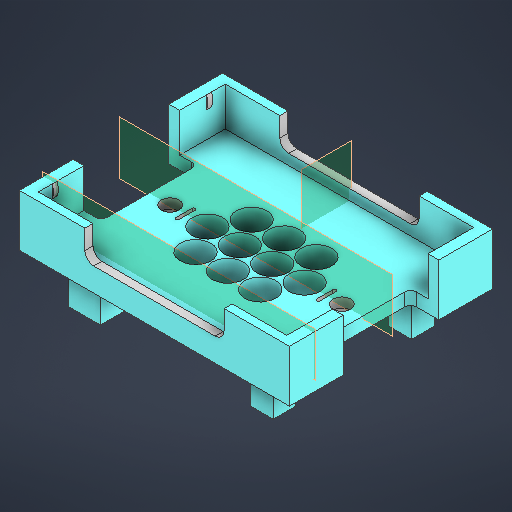
# Autodesk Inventor part: PILLARSCELLCASE18650
Saved by Autodesk Inventor 2026.2 (Build 302298000, 298)
## iProperties
Created: 2024-11-21
Part Number: PILLARSCELLCASE18650
Material: Generic
Document SubType Name: Modeling
Designer: cbast
Density: 1 g/cm^3
Appearance: Default
Mass: 190.937 g
Surface Area: 666.623 cm^2
Volume: 190.937 cm^3
Author: cbast
## iProperties of the stored document BatteryCasev1_3DPrint.ipt
Created: 2025-01-30
Part Number: BatteryCasev1_3DPrint
Material: Generic
Document SubType Name: Modeling
Designer: cbast
Density: 1 g/cm^3
Appearance: Default
Author: cbast
Autodesk Inventor part; units mm, degrees
(part 1 of 2)
ref_plane "YZ Plane" through (0, 0, 0) normal (1, 0, 0) x (0, 1, 0)
ref_plane "XZ Plane" through (0, 0, 0) normal (0, 1, 0) x (-1, 0, 0)
ref_plane "XY Plane" through (0, 0, 0) normal (0, 0, 1) x (1, 0, 0)
sketch "Sketch1" plane through (0, 0, 0) normal (0, 1, 0) x (-1, 0, 0)
  circle A0 centre (0, 0) radius 9.5
  circle A1 centre (20, 0) radius 9.5
  circle A2 centre (-20, 0) radius 9.5
  circle A3 centre (-10, 17.3205) radius 9.5
  circle A4 centre (10, 17.3205) radius 9.5
  circle A5 centre (30, 17.3205) radius 9.5
  circle A6 centre (10, -17.3205) radius 9.5
  circle A7 centre (30, -17.3205) radius 9.5
  circle A8 centre (-10, -17.3205) radius 9.5
  circle A9 centre (40, 0) radius 9.5
  line L0 (0, 0) -> (-32.9562, 0) construction
  line L1 (-32.9562, 0) -> (61.076, 0) construction
  circle A10 centre (0, 0) radius 10.5 construction
  circle A11 centre (-20, 0) radius 10.5 construction
  circle A12 centre (-10, -17.3205) radius 10.5 construction
  circle A13 centre (10, -17.3205) radius 10.5 construction
  circle A14 centre (30, -17.3205) radius 10.5 construction
  circle A15 centre (40, 0) radius 10.5 construction
  circle A16 centre (20, 0) radius 10.5 construction
  circle A17 centre (30, 17.3205) radius 10.5 construction
  circle A18 centre (10, 17.3205) radius 10.5 construction
  circle A19 centre (-10, 17.3205) radius 10.5 construction
  circle A20 centre (40, 0) radius 11.5 construction
  circle A21 centre (30, -17.3205) radius 11.5 construction
  circle A22 centre (10, -17.3205) radius 11.5 construction
  circle A23 centre (-10, -17.3205) radius 11.5 construction
  circle A24 centre (-20, 0) radius 11.5 construction
  circle A25 centre (-10, 17.3205) radius 11.5 construction
  circle A26 centre (10, 17.3205) radius 11.5 construction
  circle A27 centre (30, 17.3205) radius 11.5 construction
  circle A28 centre (0, 0) radius 11.5 construction
  circle A29 centre (20, 0) radius 11.5 construction
  arc A30 (39.9181, -11.4997) -> (39.9181, 11.4997) centre (39.9181, 0) ccw
  arc A31 (39.9181, 11.4997) -> (20, 22.9994) centre (30, 17.3205) ccw
  arc A32 (20, 22.9994) -> (0, 22.9994) centre (10, 17.3205) ccw
  arc A33 (0, 22.9994) -> (-19.9181, 11.4997) centre (-10, 17.3205) ccw
  arc A34 (-19.9181, 11.4997) -> (-19.9181, -11.4997) centre (-20, 0) ccw
  arc A35 (-19.9181, -11.4997) -> (0, -22.9994) centre (-10, -17.3205) ccw
  arc A36 (0, -22.9994) -> (20, -22.9994) centre (10, -17.3205) ccw
  arc A37 (20, -22.9994) -> (39.9181, -11.4997) centre (30, -17.3205) ccw
  point P0 (28.893, 7.4235)
  dimension "d0" = 19
  dimension "d2" = 19
  dimension "d4" = 19
  dimension "d6" = 19
  dimension "d8" = 19
  dimension "d10" = 19
  dimension "d11" = 19
  dimension "d13" = 19
  dimension "d14" = 19
  dimension "d53" = 19
  dimension "d91" = 1
  dimension "d144" = 21
  dimension "d145" = 21
  dimension "d146" = 21
  dimension "d147" = 21
  dimension "d148" = 21
  dimension "d149" = 21
  dimension "d150" = 21
  dimension "d151" = 21
  dimension "d152" = 21
  dimension "d153" = 21
  dimension "d154" = 23
  dimension "d155" = 23
  dimension "d156" = 23
  dimension "d157" = 23
  dimension "d158" = 23
  dimension "d159" = 23
  dimension "d160" = 23
  dimension "d161" = 23
  dimension "d162" = 23
  dimension "d163" = 23
  constraints: 38 centre point, 32 point on circle, 22 coincident, 16 tangent, 9 concentric, 4 end point, 2 point on line, 1 horizontal
  measures "d0" diameter of A0
  measures "d2" diameter of A1
  measures "d4" diameter of A2
  measures "d6" diameter of A3
  measures "d8" diameter of A4
  measures "d10" diameter of A5
  measures "d11" diameter of A6
  measures "d13" diameter of A7
  measures "d14" diameter of A8
  measures "d53" diameter of A9
  measures "d144" diameter of A10
  measures "d145" diameter of A11
  measures "d146" diameter of A12
  measures "d147" diameter of A13
  measures "d148" diameter of A14
  measures "d149" diameter of A15
  measures "d150" diameter of A16
  measures "d151" diameter of A17
  measures "d152" diameter of A18
  measures "d153" diameter of A19
  measures "d154" diameter of A20
  measures "d155" diameter of A21
  measures "d156" diameter of A22
  measures "d157" diameter of A23
  measures "d158" diameter of A24
  measures "d159" diameter of A25
  measures "d160" diameter of A26
  measures "d161" diameter of A27
  measures "d162" diameter of A28
  measures "d163" diameter of A29
extrude "Extrusion1" add sketch "Sketch1" along normal blind 15
sketch "Sketch4" plane through (0, 15, 0) normal (0, 1, 0) x (1, 0, 0)
  circle A0 centre (-30, 17.3205) radius 9.5 projected
  circle A1 centre (-40, 0) radius 9.5 projected
  circle A2 centre (-40, 0) radius 9.5 projected
  circle A3 centre (10, 17.3205) radius 9.5 projected
  circle A4 centre (-30, 17.3205) radius 9.5 projected
  circle A5 centre (-10, 17.3205) radius 9.5 projected
  circle A6 centre (-30, -17.3205) radius 9.5 projected
  circle A7 centre (-10, -17.3205) radius 9.5 projected
  circle A8 centre (10, -17.3205) radius 9.5 projected
  circle A9 centre (20, 0) radius 9.5 projected
  circle A10 centre (-20, 0) radius 9.5 projected
  circle A11 centre (0, 0) radius 9.5 projected
  line L0 (0, 0) -> (-10, 0) construction
  line L1 (-86.7, 57.7) -> (66.7, 57.7)
  line L2 (66.7, 57.7) -> (66.7, -57.7)
  line L3 (66.7, -57.7) -> (-86.7, -57.7)
  line L4 (-86.7, -57.7) -> (-86.7, 57.7)
  line L5 (-86.7, 57.7) -> (66.7, -57.7) construction
  line L6 (66.7, 57.7) -> (-86.7, -57.7) construction
  arc A12 (0, 22.9994) -> (-20, 22.9994) centre (-10, 17.3205) ccw projected
  arc A13 (19.9181, 11.4997) -> (0, 22.9994) centre (10, 17.3205) ccw projected
  arc A14 (19.9181, -11.4997) -> (19.9181, 11.4997) centre (20, 0) ccw projected
  arc A15 (0, -22.9994) -> (19.9181, -11.4997) centre (10, -17.3205) ccw projected
  arc A16 (-20, -22.9994) -> (0, -22.9994) centre (-10, -17.3205) ccw projected
  arc A17 (-39.9181, -11.4997) -> (-20, -22.9994) centre (-30, -17.3205) ccw projected
  circle A18 centre (-30, 17.3205) radius 11.5 construction
  arc A19 (-39.9181, 11.4997) -> (-39.9181, -11.4997) centre (-39.9181, 0) ccw projected
  arc A20 (-20, 22.9994) -> (-39.9181, 11.4997) centre (-30, 17.3205) ccw projected
  arc A21 (0, 22.9994) -> (-20, 22.9994) centre (-10, 17.3205) ccw
  arc A22 (19.9181, 11.4997) -> (0, 22.9994) centre (10, 17.3205) ccw
  arc A23 (19.9181, -11.4997) -> (19.9181, 11.4997) centre (20, 0) ccw
  arc A24 (0, -22.9994) -> (19.9181, -11.4997) centre (10, -17.3205) ccw
  arc A25 (-20, -22.9994) -> (0, -22.9994) centre (-10, -17.3205) ccw
  arc A26 (-39.9181, -11.4997) -> (-20, -22.9994) centre (-30, -17.3205) ccw
  arc A27 (-39.9181, 11.4997) -> (-39.9181, -11.4997) centre (-39.9181, 0) ccw
  arc A28 (-20, 22.9994) -> (-39.9181, 11.4997) centre (-30, 17.3205) ccw
  line L7 (-10.5, 0) -> (-9.5, 0) construction
  point P0 (-17.0502, -21.4927)
  point P1 (-17.0502, -11.5134)
  point P2 (-17.0502, -8.8009)
  point P3 (-17.0502, 8.8009)
  point P4 (-17.0502, 11.5134)
  point P5 (-17.0502, 21.4927)
  point P6 (-2.0059, 21.4927)
  point P7 (-2.0059, -11.5134)
  point P8 (-2.0059, -8.8009)
  point P9 (-2.0059, 8.8009)
  point P10 (-2.0059, 11.5134)
  point P11 (-2.0059, -21.4927)
  point P12 (-86.7, 0)
  point P13 (66.7, 0)
  dimension "d104" = 153.4
  dimension "d164" = 115.4
  dimension "d233" = 76.7
  dimension "d234" = 76.7
  constraints: 16 end point, 16 point on circle, 8 centre point, 8 concentric, 5 midpoint, 2 horizontal, 2 parallel, 1 perpendicular, 1 point on line, 4 other
  measures "d104" distance of L2.end L3.end
  measures "d164" distance of L1.end L2.end
  measures "d233" distance of point (-86.7, 0) L0.end
  measures "d234" distance of point (66.7, 0) L0.end
extrude "Extrusion7" add sketch "Sketch4" against normal blind 8 contours L1 L2 L3 L4
sketch "Sketch5" plane through (0, 15, 0) normal (0, 1, 0) x (1, 0, 0)
  line L0 (-86.7, -57.7) -> (66.7, -57.7) projected
  line L1 (66.7, -57.7) -> (66.7, 57.7) projected
  line L2 (66.7, 57.7) -> (-86.7, 57.7) projected
  line L3 (-86.7, 57.7) -> (-86.7, -57.7) projected
  circle A0 centre (-40, 0) radius 9.5 projected
  circle A1 centre (10, 17.3205) radius 9.5 projected
  circle A2 centre (-30, 17.3205) radius 9.5 projected
  circle A3 centre (-10, 17.3205) radius 9.5 projected
  circle A4 centre (-30, -17.3205) radius 9.5 projected
  circle A5 centre (-10, -17.3205) radius 9.5 projected
  circle A6 centre (10, -17.3205) radius 9.5 projected
  circle A7 centre (20, 0) radius 9.5 projected
  circle A8 centre (-20, 0) radius 9.5 projected
  circle A9 centre (0, 0) radius 9.5 projected
  line L4 (-86.7, 57.7) -> (66.7, 57.7)
  line L5 (66.7, 57.7) -> (66.7, -57.7)
  line L6 (66.7, -57.7) -> (-86.7, -57.7)
  line L7 (-86.7, -57.7) -> (-86.7, 57.7)
  line L8 (-93.3464, -62.7) -> (73.3464, -62.7)
  line L9 (73.3464, -62.7) -> (73.3464, 62.7)
  line L10 (73.3464, 62.7) -> (-93.3464, 62.7)
  line L11 (-93.3464, 62.7) -> (-93.3464, -62.7)
  line L12 (-93.3464, -62.7) -> (73.3464, 62.7) construction
  line L13 (73.3464, -62.7) -> (-93.3464, 62.7) construction
  point P0 (66.922, -57.45)
  point P1 (-10, 0)
  dimension "d169" = 5
  dimension "d170" = 6.6464
  dimension "d171" = 166.6929
  dimension "d172" = 125.4
  dimension "d221" = 6.6464
  constraints: 20 end point, 4 parallel, 4 point on line, 2 horizontal, 2 midpoint, 2 perpendicular
  measures "d169" distance between parallel lines of L10 L4
  measures "d170" distance between parallel lines of L9 L5
  measures "d171" distance of L9.end L10.end
  measures "d172" distance of L10.end L8.start
  measures "d221" distance between parallel lines of L3 L11
extrude "Extrusion8" add sketch "Sketch5" along normal blind 24 and the other way blind 8 contours L11 L10 L9 L8
sketch "Sketch6" plane through (0, 15, 0) normal (0, 1, 0) x (1, 0, 0)
  line L0 (59.472, 57.1514) -> (59.472, 25.95) construction
  line L1 (59.472, 25.95) -> (66.7, 25.95) construction
  line L2 (-79.472, -57.7) -> (-79.472, -25.95) construction
  line L3 (-79.472, -25.95) -> (-86.7, -25.95) construction
  circle A0 centre (59.472, 25.95) radius 3.615
  circle A1 centre (59.472, -25.95) radius 3.615
  circle A2 centre (-79.472, -25.95) radius 3.615
  circle A3 centre (-79.472, 25.95) radius 3.615
  line L4 (73.3464, -62.7) -> (73.3464, 62.7) projected
  line L5 (73.3464, 62.7) -> (-93.3464, 62.7) projected
  line L6 (-93.3464, 62.7) -> (-93.3464, -62.7) projected
  line L7 (-93.3464, -62.7) -> (73.3464, -62.7) projected
  line L8 (-86.7, -57.7) -> (-86.7, 57.7) projected
  line L9 (-86.7, 57.7) -> (66.7, 57.7) projected
  line L10 (66.7, 57.7) -> (66.7, -57.7) projected
  line L11 (66.7, -57.7) -> (-86.7, -57.7) projected
  line L12 (-86.7, -57.7) -> (66.7, -57.7) projected
  line L13 (66.7, -57.7) -> (66.7, 57.7) projected
  line L14 (66.7, 57.7) -> (-86.7, 57.7) projected
  line L15 (-86.7, 57.7) -> (-86.7, -57.7) projected
  circle A4 centre (-40, 0) radius 9.5 projected
  circle A5 centre (10, 17.3205) radius 9.5 projected
  circle A6 centre (-30, 17.3205) radius 9.5 projected
  circle A7 centre (-10, 17.3205) radius 9.5 projected
  circle A8 centre (-30, -17.3205) radius 9.5 projected
  circle A9 centre (-10, -17.3205) radius 9.5 projected
  circle A10 centre (10, -17.3205) radius 9.5 projected
  circle A11 centre (20, 0) radius 9.5 projected
  circle A12 centre (-20, 0) radius 9.5 projected
  circle A13 centre (0, 0) radius 9.5 projected
  line L16 (-86.7, 57.7) -> (66.7, 57.7)
  line L17 (66.7, 57.7) -> (66.7, -57.7)
  line L18 (66.7, -57.7) -> (-86.7, -57.7)
  line L19 (-86.7, -57.7) -> (-86.7, 57.7)
  dimension "d123" = 7.23
  dimension "d124" = 7.23
  dimension "d125" = 7.23
  dimension "d140" = 7.23
  dimension "d179" = 31.75
  dimension "d180" = 7.228
  dimension "d181" = 7.228
  dimension "d182" = 31.75
  dimension "d183" = 31.75
  dimension "d184" = 7.228
  dimension "d185" = 7.228
  dimension "d186" = 31.75
  constraints: 16 end point, 4 centre point, 2 coincident, 2 parallel, 1 horizontal, 1 perpendicular
  measures "d123" diameter of A0
  measures "d124" diameter of A1
  measures "d125" diameter of A2
  measures "d140" diameter of A3
  measures "d179" distance from line of A3.centre L16
  measures "d180" distance from line of A3.centre L15
  measures "d181" distance from line of A2.centre L8
  measures "d182" distance from line of L2.end L18
  measures "d183" distance from line of L12 A1.centre
  measures "d184" distance from line of L17 A1.centre
  measures "d185" distance from line of L17 L0.end
  measures "d186" distance from line of L16 L0.end
extrude "Extrusion6" cut sketch "Sketch6" against normal through all contours A0 | A1 | A2 | A3
sketch "Sketch7" plane through (-93.3464, 7, 62.7) normal (-1, 0, 0) x (0, 0, 1)
  line L0 (-120.4, 8) -> (-5, 8) projected
  line L1 (0, 0) -> (-125.4, 0) projected
  line L2 (-125.4, 32) -> (0, 32) projected
  line L3 (-92.265, 8) -> (-85.035, 8) projected
  line L4 (-40.365, 8) -> (-33.135, 8) projected
  line L5 (-92.265, 8) -> (-33.135, 8)
  line L6 (-33.135, 8) -> (-33.135, 32)
  line L7 (-33.135, 32) -> (-92.265, 32)
  line L8 (-92.265, 32) -> (-92.265, 8)
  point P0 (-62.7, -7)
  point P1 (-92.265, 32)
  constraints: 8 end point, 2 parallel, 1 horizontal, 1 perpendicular, 1 point on line
extrude "Extrusion9" cut sketch "Sketch7" against normal through all
sketch "Sketch10" plane through (0, 7, 0) normal (0, -1, 0) x (1, 0, 0)
  circle A0 centre (-79.472, 25.95) radius 3.615 projected
  circle A1 centre (59.472, 25.95) radius 3.615 projected
  circle A2 centre (-79.472, -25.95) radius 3.615 projected
  circle A3 centre (59.472, -25.95) radius 3.615 projected
  line L0 (73.3464, -62.7) -> (73.3464, 62.7) projected
  line L1 (73.3464, 62.7) -> (-93.3464, 62.7) projected
  line L2 (-93.3464, 62.7) -> (-93.3464, -62.7) projected
  line L3 (-93.3464, -62.7) -> (73.3464, -62.7) projected
  arc A4 (-39.9181, -11.4997) -> (-20, -22.9994) centre (-30, -17.3205) ccw projected
  arc A5 (-39.9181, 11.4997) -> (-39.9181, -11.4997) centre (-39.9181, 0) ccw projected
  arc A6 (-20, 22.9994) -> (-39.9181, 11.4997) centre (-30, 17.3205) ccw projected
  arc A7 (0, 22.9994) -> (-20, 22.9994) centre (-10, 17.3205) ccw projected
  arc A8 (19.9181, 11.4997) -> (0, 22.9994) centre (10, 17.3205) ccw projected
  arc A9 (19.9181, -11.4997) -> (19.9181, 11.4997) centre (20, 0) ccw projected
  arc A10 (0, -22.9994) -> (19.9181, -11.4997) centre (10, -17.3205) ccw projected
  arc A11 (-20, -22.9994) -> (0, -22.9994) centre (-10, -17.3205) ccw projected
  line L4 (-93.3464, 62.7) -> (-63.3464, 62.7) construction
  line L5 (-93.3464, 62.7) -> (-93.3464, 42.7) construction
  line L6 (-93.3464, 42.7) -> (-63.3464, 42.7) construction
  line L7 (-73.3464, 52.7) -> (-53.3464, 52.7)
  line L8 (-53.3464, 52.7) -> (-53.3464, 32.7)
  line L9 (-53.3464, 32.7) -> (-73.3464, 32.7)
  line L10 (-73.3464, 32.7) -> (-73.3464, 52.7)
  line L11 (-73.3464, 52.7) -> (-53.3464, 32.7) construction
  line L12 (-53.3464, 52.7) -> (-73.3464, 32.7) construction
  line L13 (-70.8464, 50.2) -> (-55.8464, 50.2)
  line L14 (-55.8464, 50.2) -> (-55.8464, 35.2)
  line L15 (-55.8464, 35.2) -> (-70.8464, 35.2)
  line L16 (-70.8464, 35.2) -> (-70.8464, 50.2)
  line L17 (-70.8464, 50.2) -> (-55.8464, 35.2) construction
  line L18 (-55.8464, 50.2) -> (-70.8464, 35.2) construction
  line L19 (-93.3464, 0) -> (73.3464, 0) construction
  line L20 (-73.3464, -52.7) -> (-53.3464, -52.7)
  line L21 (-53.3464, -52.7) -> (-53.3464, -32.7)
  line L22 (-53.3464, -32.7) -> (-73.3464, -32.7)
  line L23 (-73.3464, -32.7) -> (-73.3464, -52.7)
  line L24 (-73.3464, -52.7) -> (-53.3464, -32.7) construction
  line L25 (-53.3464, -52.7) -> (-73.3464, -32.7) construction
  line L26 (-70.8464, -50.2) -> (-55.8464, -50.2)
  line L27 (-55.8464, -50.2) -> (-55.8464, -35.2)
  line L28 (-55.8464, -35.2) -> (-70.8464, -35.2)
  line L29 (-70.8464, -35.2) -> (-70.8464, -50.2)
  line L30 (-70.8464, -50.2) -> (-55.8464, -35.2) construction
  line L31 (-55.8464, -50.2) -> (-70.8464, -35.2) construction
  line L32 (73.3464, 62.7) -> (43.3464, 62.7) construction
  line L33 (43.3464, 62.7) -> (43.3464, 42.7) construction
  line L34 (36.3464, 49.7) -> (50.3464, 49.7)
  line L35 (50.3464, 49.7) -> (50.3464, 35.7)
  line L36 (50.3464, 35.7) -> (36.3464, 35.7)
  line L37 (36.3464, 35.7) -> (36.3464, 49.7)
  line L38 (36.3464, 49.7) -> (50.3464, 35.7) construction
  line L39 (50.3464, 49.7) -> (36.3464, 35.7) construction
  line L40 (36.3464, -49.7) -> (50.3464, -49.7)
  line L41 (50.3464, -49.7) -> (50.3464, -35.7)
  line L42 (50.3464, -35.7) -> (36.3464, -35.7)
  line L43 (36.3464, -35.7) -> (36.3464, -49.7)
  line L44 (36.3464, -49.7) -> (50.3464, -35.7) construction
  line L45 (50.3464, -49.7) -> (36.3464, -35.7) construction
  line L46 (43.3464, -42.7) -> (43.3464, -62.7) construction
  line L47 (43.3464, -42.7) -> (73.3464, -42.7) construction
  line L48 (-63.3464, -42.7) -> (-63.3464, -62.7) construction
  line L49 (-63.3464, -42.7) -> (-93.3464, -42.7) construction
  point P0 (0, 0)
  dimension "d209" = 30
  dimension "d210" = 20
  dimension "d211" = 20
  dimension "d212" = 20
  dimension "d213" = 15
  dimension "d214" = 15
  dimension "d215" = 30
  dimension "d216" = 20
  dimension "d217" = 14
  dimension "d218" = 14
  dimension "d224" = 30
  dimension "d225" = 30
  dimension "d226" = 20
  dimension "d227" = 20
  constraints: 92 end point, 14 symmetric about line, 8 midpoint, 8 point on line, 7 parallel, 6 perpendicular, 4 horizontal
  measures "d209" distance of L1.end L4.end
  measures "d210" distance of L1.end L5.end
  measures "d211" distance of L8.end L9.end
  measures "d212" distance of L7.end L8.end
  measures "d213" distance of L14.end L15.end
  measures "d214" distance of L13.end L14.end
  measures "d215" distance of L0.end L32.end
  measures "d216" distance of L32.end L33.end
  measures "d217" distance of L35.end L36.end
  measures "d218" distance of L34.end L35.end
  measures "d224" distance of L48.start L49.end
  measures "d225" distance of L46.start L47.end
  measures "d226" distance of L46.start L46.end
  measures "d227" distance of L48.start L48.end
extrude "Extrusion11" add sketch "Sketch10" along normal blind 25 contours L7 L8 L9 L10 | L23 L22 L21 L20 | L34 L35 L36 L37 | L43 L42 L41 L40
sketch "Sketch11" plane through (0, 7, 0) normal (0, -1, 0) x (1, 0, 0)
  line L0 (-70.8464, 50.2) -> (-70.8464, 35.2) projected
  line L1 (-70.8464, 35.2) -> (-55.8464, 35.2) projected
  line L2 (-55.8464, 35.2) -> (-55.8464, 50.2) projected
  line L3 (-55.8464, 50.2) -> (-70.8464, 50.2) projected
  line L4 (-70.8464, 50.2) -> (-55.8464, 50.2)
  line L5 (-55.8464, 50.2) -> (-55.8464, 35.2)
  line L6 (-55.8464, 35.2) -> (-70.8464, 35.2)
  line L7 (-70.8464, 35.2) -> (-70.8464, 50.2)
  line L8 (-55.8464, -35.2) -> (-70.8464, -35.2) projected
  line L9 (-70.8464, -35.2) -> (-70.8464, -50.2) projected
  line L10 (-70.8464, -50.2) -> (-55.8464, -50.2) projected
  line L11 (-55.8464, -50.2) -> (-55.8464, -35.2) projected
  line L12 (-70.8464, -35.2) -> (-55.8464, -35.2)
  line L13 (-55.8464, -35.2) -> (-55.8464, -50.2)
  line L14 (-55.8464, -50.2) -> (-70.8464, -50.2)
  line L15 (-70.8464, -50.2) -> (-70.8464, -35.2)
  point P0 (0, 0)
  constraints: 16 end point, 4 parallel, 2 horizontal, 2 perpendicular
extrude "Extrusion12" add sketch "Sketch11" along normal up to surface (12.5 mm away)
sketch "Sketch13" plane through (0, 7, 0) normal (0, -1, 0) x (1, 0, 0)
  line L0 (36.3464, 35.7) -> (36.3464, 49.7) projected
  line L1 (36.3464, 49.7) -> (50.3464, 49.7) projected
  line L2 (50.3464, 49.7) -> (50.3464, 35.7) projected
  line L3 (50.3464, 35.7) -> (36.3464, 35.7) projected
  line L4 (-73.3464, -32.7) -> (-53.3464, -32.7) projected
  line L5 (-53.3464, -32.7) -> (-53.3464, -52.7) projected
  line L6 (-53.3464, -52.7) -> (-73.3464, -52.7) projected
  line L7 (-73.3464, -52.7) -> (-73.3464, -32.7) projected
  line L8 (36.3464, -49.7) -> (36.3464, -35.7) projected
  line L9 (36.3464, -35.7) -> (50.3464, -35.7) projected
  line L10 (50.3464, -35.7) -> (50.3464, -49.7) projected
  line L11 (50.3464, -49.7) -> (36.3464, -49.7) projected
  line L12 (-73.3464, 32.7) -> (-73.3464, 52.7) projected
  line L13 (-73.3464, 52.7) -> (-53.3464, 52.7) projected
  line L14 (-53.3464, 52.7) -> (-53.3464, 32.7) projected
  line L15 (-53.3464, 32.7) -> (-73.3464, 32.7) projected
  circle A0 centre (-79.472, 25.95) radius 3.615 projected
  circle A1 centre (59.472, 25.95) radius 3.615 projected
  circle A2 centre (-79.472, -25.95) radius 3.615 projected
  circle A3 centre (59.472, -25.95) radius 3.615 projected
  line L16 (73.3464, -62.7) -> (73.3464, 62.7) projected
  line L17 (73.3464, 62.7) -> (-93.3464, 62.7) projected
  line L18 (-93.3464, 62.7) -> (-93.3464, -62.7) projected
  line L19 (-93.3464, -62.7) -> (73.3464, -62.7) projected
  arc A4 (-39.9181, -11.4997) -> (-20, -22.9994) centre (-30, -17.3205) ccw projected
  arc A5 (-39.9181, 11.4997) -> (-39.9181, -11.4997) centre (-39.9181, 0) ccw projected
  arc A6 (-20, 22.9994) -> (-39.9181, 11.4997) centre (-30, 17.3205) ccw projected
  arc A7 (0, 22.9994) -> (-20, 22.9994) centre (-10, 17.3205) ccw projected
  arc A8 (19.9181, 11.4997) -> (0, 22.9994) centre (10, 17.3205) ccw projected
  arc A9 (19.9181, -11.4997) -> (19.9181, 11.4997) centre (20, 0) ccw projected
  arc A10 (0, -22.9994) -> (19.9181, -11.4997) centre (10, -17.3205) ccw projected
  arc A11 (-20, -22.9994) -> (0, -22.9994) centre (-10, -17.3205) ccw projected
  line L20 (-93.3464, 29.565) -> (-75.857, 29.565)
  line L21 (-75.857, 29.565) -> (-75.857, -29.565)
  line L22 (-75.857, -29.565) -> (-93.3464, -29.565)
  line L23 (-93.3464, -29.565) -> (-93.3464, 29.565)
  line L24 (-10, 27.2798) -> (-10, -25.95) construction
  line L25 (73.3464, 29.565) -> (55.857, 29.565)
  line L26 (55.857, 29.565) -> (55.857, -29.565)
  line L27 (55.857, -29.565) -> (73.3464, -29.565)
  circle A12 centre (-79.472, -25.95) radius 3.615 projected
  line L28 (-86.7, 29.565) -> (-86.7, 57.7) projected
  line L29 (-86.7, 57.7) -> (66.7, 57.7) projected
  line L30 (66.7, 57.7) -> (66.7, 29.565) projected
  line L31 (66.7, 29.565) -> (73.3464, 29.565) projected
  line L32 (73.3464, -29.565) -> (73.3464, 29.565) projected
  line L33 (66.7, -29.565) -> (73.3464, -29.565) projected
  line L34 (66.7, -29.565) -> (66.7, -57.7) projected
  line L35 (66.7, -57.7) -> (-86.7, -57.7) projected
  line L36 (-86.7, -57.7) -> (-86.7, -29.565) projected
  line L37 (-93.3464, -29.565) -> (-86.7, -29.565) projected
  line L38 (-93.3464, 29.565) -> (-93.3464, -29.565) projected
  line L39 (-93.3464, 29.565) -> (-86.7, 29.565) projected
  circle A13 centre (59.472, -25.95) radius 3.615 projected
  circle A14 centre (-79.472, 25.95) radius 3.615 projected
  circle A15 centre (-40, 0) radius 9.5 projected
  circle A16 centre (10, -17.3205) radius 9.5 projected
  circle A17 centre (-30, -17.3205) radius 9.5 projected
  circle A18 centre (-10, -17.3205) radius 9.5 projected
  circle A19 centre (-30, 17.3205) radius 9.5 projected
  circle A20 centre (-10, 17.3205) radius 9.5 projected
  circle A21 centre (10, 17.3205) radius 9.5 projected
  circle A22 centre (20, 0) radius 9.5 projected
  circle A23 centre (-20, 0) radius 9.5 projected
  circle A24 centre (0, 0) radius 9.5 projected
  circle A25 centre (59.472, 25.95) radius 3.615 projected
  line L40 (-10.5, 0) -> (-9.5, 0) construction
  point P0 (59.472, -29.565)
  point P1 (59.472, 29.565)
  point P2 (55.857, 25.95)
  point P3 (55.857, -25.95)
  point P4 (-79.472, -29.565)
  point P5 (-75.857, -25.95)
  point P6 (-75.857, 25.95)
  point P7 (-79.472, 29.565)
  dimension "d235" = 17.4895
  dimension "d236" = 17.4895
  constraints: 18 end point, 4 symmetric about line, 2 horizontal, 2 horizontal alignment, 2 parallel, 1 perpendicular, 1 point on line, 1 vertical, 2 other
  measures "d235" distance between parallel lines of L21 L18
  measures "d236" distance between parallel lines of L16 L26
extrude "Extrusion14" cut sketch "Sketch13" against normal blind 10 contours L21 A2 L22 L18 L20 A0 | L25 L16 L27 A3 L26 A1
sketch "Sketch15" plane through (0, 7, 0) normal (0, -1, 0) x (1, 0, 0)
  line L0 (-39.8605, 53.1473) -> (15.842, 53.1473) construction
  line L1 (15.842, 53.1473) -> (15.842, 30.1509) construction
  line L2 (15.842, 30.1509) -> (-39.8605, 30.1509) construction
  line L3 (-39.8605, 30.1509) -> (-39.8605, 53.1473) construction
  line L4 (-27.8722, 48.7866) -> (-30.2445, 48.7866)
  line L5 (-30.2445, 48.7866) -> (-30.6581, 47.8297)
  spline S0 degree 2 poles (-30.6581, 47.8297) (-30.8126, 47.4709) (-30.8126, 47.2965) knots 0 0 0 1 1 1
  spline S1 degree 2 poles (-30.8126, 47.2965) (-30.8126, 47.157) (-30.5435, 46.9427) (-30.1049, 46.9128) knots 0 0 0 1 2 2 2
  line L6 (-30.1049, 46.9128) -> (-30.1049, 46.7483)
  line L7 (-30.1049, 46.7483) -> (-32.0286, 46.7483)
  line L8 (-32.0286, 46.7483) -> (-32.0286, 46.9128)
  spline S2 degree 2 poles (-32.0286, 46.9128) (-31.6449, 46.9825) (-31.5352, 47.0872) knots 0 0 0 1 1 1
  spline S3 degree 2 poles (-31.5352, 47.0872) (-31.306, 47.3065) (-31.0269, 47.9693) knots 0 0 0 1 1 1
  line L9 (-31.0269, 47.9693) -> (-28.874, 52.9878)
  line L10 (-28.874, 52.9878) -> (-28.7145, 52.9878)
  line L11 (-28.7145, 52.9878) -> (-26.5914, 47.9145)
  spline S4 degree 2 poles (-26.5914, 47.9145) (-26.3373, 47.3015) (-25.9186, 46.9377) (-25.5449, 46.9128) knots 0 0 0 1 2 2 2
  line L12 (-25.5449, 46.9128) -> (-25.5449, 46.7483)
  line L13 (-25.5449, 46.7483) -> (-27.952, 46.7483)
  line L14 (-27.952, 46.7483) -> (-27.952, 46.9128)
  spline S5 degree 2 poles (-27.952, 46.9128) (-27.5882, 46.9327) (-27.329, 47.137) (-27.329, 47.2865) knots 0 0 0 1 2 2 2
  spline S6 degree 2 poles (-27.329, 47.2865) (-27.329, 47.4859) (-27.5084, 47.9145) knots 0 0 0 1 1 1
  line L15 (-27.5084, 47.9145) -> (-27.8722, 48.7866)
  line L16 (-28.0118, 49.1205) -> (-29.0384, 51.5874)
  line L17 (-29.0384, 51.5874) -> (-30.1049, 49.1205)
  line L18 (-30.1049, 49.1205) -> (-28.0118, 49.1205)
  line L19 (-19.2156, 46.7483) -> (-20.8453, 46.7483)
  line L20 (-20.8453, 46.7483) -> (-22.9135, 49.5989)
  spline S7 degree 2 poles (-22.9135, 49.5989) (-23.1427, 49.589) (-23.2823, 49.589) knots 0 0 0 1 1 1
  spline S8 degree 2 poles (-23.2823, 49.589) (-23.3421, 49.589) (-23.4767, 49.594) (-23.5464, 49.5989) knots 0 0 0 1 2 2 2
  line L21 (-23.5464, 49.5989) -> (-23.5464, 47.8297)
  spline S9 degree 2 poles (-23.5464, 47.8297) (-23.5464, 47.2516) (-23.4218, 47.1121) knots 0 0 0 1 1 1
  spline S10 degree 2 poles (-23.4218, 47.1121) (-23.2524, 46.9128) (-22.9135, 46.9128) knots 0 0 0 1 1 1
  line L22 (-22.9135, 46.9128) -> (-22.6743, 46.9128)
  line L23 (-22.6743, 46.9128) -> (-22.6743, 46.7483)
  line L24 (-22.6743, 46.7483) -> (-25.2807, 46.7483)
  line L25 (-25.2807, 46.7483) -> (-25.2807, 46.9128)
  line L26 (-25.2807, 46.9128) -> (-25.0515, 46.9128)
  spline S11 degree 2 poles (-25.0515, 46.9128) (-24.6677, 46.9128) (-24.5033, 47.1669) knots 0 0 0 1 1 1
  spline S12 degree 2 poles (-24.5033, 47.1669) (-24.4086, 47.3065) (-24.4086, 47.8297) knots 0 0 0 1 1 1
  line L27 (-24.4086, 47.8297) -> (-24.4086, 51.7668)
  spline S13 degree 2 poles (-24.4086, 51.7668) (-24.4086, 52.3449) (-24.5332, 52.4845) knots 0 0 0 1 1 1
  spline S14 degree 2 poles (-24.5332, 52.4845) (-24.7076, 52.6838) (-25.0515, 52.6838) knots 0 0 0 1 1 1
  line L28 (-25.0515, 52.6838) -> (-25.2807, 52.6838)
  line L29 (-25.2807, 52.6838) -> (-25.2807, 52.8483)
  line L30 (-25.2807, 52.8483) -> (-23.063, 52.8483)
  spline S15 degree 2 poles (-23.063, 52.8483) (-22.0912, 52.8483) (-21.1692, 52.5642) (-20.5263, 51.8067) (-20.5263, 51.2784) knots 0 0 0 1 2 3 3 3
  spline S16 degree 2 poles (-20.5263, 51.2784) (-20.5263, 50.7153) (-21.2589, 49.888) (-22.0314, 49.7186) knots 0 0 0 1 2 2 2
  line L31 (-22.0314, 49.7186) -> (-20.7655, 47.9693)
  spline S17 degree 2 poles (-20.7655, 47.9693) (-20.332, 47.3663) (-19.714, 46.9676) (-19.2156, 46.9128) knots 0 0 0 1 2 2 2
  line L32 (-19.2156, 46.9128) -> (-19.2156, 46.7483)
  spline S18 degree 2 poles (-23.5464, 49.883) (-23.4617, 49.883) (-23.3371, 49.878) (-23.2972, 49.878) knots 0 0 0 1 2 2 2
  spline S19 degree 2 poles (-23.2972, 49.878) (-22.4351, 49.878) (-21.5579, 50.6355) (-21.5579, 51.2186) knots 0 0 0 1 2 2 2
  spline S20 degree 2 poles (-21.5579, 51.2186) (-21.5579, 51.7918) (-22.2656, 52.5044) (-22.8487, 52.5044) knots 0 0 0 1 2 2 2
  spline S21 degree 2 poles (-22.8487, 52.5044) (-23.1079, 52.5044) (-23.5464, 52.4197) knots 0 0 0 1 1 1
  line L33 (-23.5464, 52.4197) -> (-23.5464, 49.883)
  line L34 (-13.9728, 52.8483) -> (-13.908, 51.418)
  line L35 (-13.908, 51.418) -> (-14.0775, 51.418)
  spline S22 degree 2 poles (-14.0775, 51.418) (-14.1273, 51.7918) (-14.212, 51.9562) knots 0 0 0 1 1 1
  spline S23 degree 2 poles (-14.212, 51.9562) (-14.3516, 52.2154) (-14.815, 52.4645) (-15.1938, 52.4645) knots 0 0 0 1 2 2 2
  line L36 (-15.1938, 52.4645) -> (-16.051, 52.4645)
  line L37 (-16.051, 52.4645) -> (-16.051, 47.8048)
  spline S24 degree 2 poles (-16.051, 47.8048) (-16.051, 47.2417) (-15.9314, 47.1021) knots 0 0 0 1 1 1
  spline S25 degree 2 poles (-15.9314, 47.1021) (-15.757, 46.9128) (-15.4031, 46.9128) knots 0 0 0 1 1 1
  line L38 (-15.4031, 46.9128) -> (-15.1938, 46.9128)
  line L39 (-15.1938, 46.9128) -> (-15.1938, 46.7483)
  line L40 (-15.1938, 46.7483) -> (-17.7753, 46.7483)
  line L41 (-17.7753, 46.7483) -> (-17.7753, 46.9128)
  line L42 (-17.7753, 46.9128) -> (-17.561, 46.9128)
  spline S26 degree 2 poles (-17.561, 46.9128) (-17.1723, 46.9128) (-17.0128, 47.147) knots 0 0 0 1 1 1
  spline S27 degree 2 poles (-17.0128, 47.147) (-16.9132, 47.2915) (-16.9132, 47.8048) knots 0 0 0 1 1 1
  line L43 (-16.9132, 47.8048) -> (-16.9132, 52.4645)
  line L44 (-16.9132, 52.4645) -> (-17.6458, 52.4645)
  spline S28 degree 2 poles (-17.6458, 52.4645) (-18.0744, 52.4645) (-18.2538, 52.3998) knots 0 0 0 1 1 1
  spline S29 degree 2 poles (-18.2538, 52.3998) (-18.488, 52.315) (-18.8169, 51.8316) (-18.8518, 51.418) knots 0 0 0 1 2 2 2
  line L45 (-18.8518, 51.418) -> (-19.0213, 51.418)
  line L46 (-19.0213, 51.418) -> (-18.9515, 52.8483)
  line L47 (-18.9515, 52.8483) -> (-13.9728, 52.8483)
  line L48 (-9.4377, 52.9878) -> (-9.4377, 50.8797)
  line L49 (-9.4377, 50.8797) -> (-9.6021, 50.8797)
  spline S30 degree 2 poles (-9.6021, 50.8797) (-9.6819, 51.4878) (-10.1055, 52.2054) (-10.878, 52.629) (-11.2966, 52.629) knots 0 0 0 1 2 3 3 3
  spline S31 degree 2 poles (-11.2966, 52.629) (-11.765, 52.629) (-12.378, 52.0559) (-12.378, 51.6921) knots 0 0 0 1 2 2 2
  spline S32 degree 2 poles (-12.378, 51.6921) (-12.378, 51.413) (-12.1837, 51.1837) knots 0 0 0 1 1 1
  spline S33 degree 2 poles (-12.1837, 51.1837) (-11.9046, 50.8449) (-10.853, 50.2817) knots 0 0 0 1 1 1
  spline S34 degree 2 poles (-10.853, 50.2817) (-10.0008, 49.8232) (-9.3729, 49.3348) (-9.034, 48.667) (-9.034, 48.3032) knots 0 0 0 1 2 3 3 3
  spline S35 degree 2 poles (-9.034, 48.3032) (-9.034, 47.6105) (-10.1105, 46.6087) (-10.9577, 46.6087) knots 0 0 0 1 2 2 2
  spline S36 degree 2 poles (-10.9577, 46.6087) (-11.2218, 46.6087) (-11.4561, 46.6486) knots 0 0 0 1 1 1
  spline S37 degree 2 poles (-11.4561, 46.6486) (-11.5956, 46.6735) (-12.4727, 46.9576) (-12.5923, 46.9576) knots 0 0 0 1 2 2 2
  spline S38 degree 2 poles (-12.5923, 46.9576) (-12.702, 46.9576) (-12.8365, 46.823) (-12.8664, 46.6087) knots 0 0 0 1 2 2 2
  line L50 (-12.8664, 46.6087) -> (-13.0309, 46.6087)
  line L51 (-13.0309, 46.6087) -> (-13.0309, 48.7019)
  line L52 (-13.0309, 48.7019) -> (-12.8664, 48.7019)
  spline S39 degree 2 poles (-12.8664, 48.7019) (-12.7518, 48.044) (-12.3531, 47.3912) (-11.5358, 46.9576) (-11.0524, 46.9576) knots 0 0 0 1 2 3 3 3
  spline S40 degree 2 poles (-11.0524, 46.9576) (-10.4892, 46.9576) (-9.8364, 47.5507) (-9.8364, 47.9593) knots 0 0 0 1 2 2 2
  spline S41 degree 2 poles (-9.8364, 47.9593) (-9.8364, 48.1836) (-10.0856, 48.6421) (-10.3447, 48.8414) knots 0 0 0 1 2 2 2
  spline S42 degree 2 poles (-10.3447, 48.8414) (-10.5191, 48.976) (-12.089, 49.8531) (-12.7518, 50.3764) (-13.0957, 51.0043) (-13.0957, 51.3831) knots 0 0 0 1 2 3 4 4 4
  spline S43 degree 2 poles (-13.0957, 51.3831) (-13.0957, 52.0409) (-12.084, 52.9878) (-11.3016, 52.9878) knots 0 0 0 1 2 2 2
  spline S44 degree 2 poles (-11.3016, 52.9878) (-10.8182, 52.9878) (-10.27, 52.7486) knots 0 0 0 1 1 1
  spline S45 degree 2 poles (-10.27, 52.7486) (-10.0158, 52.639) (-9.9111, 52.639) knots 0 0 0 1 1 1
  spline S46 degree 2 poles (-9.9111, 52.639) (-9.7965, 52.639) (-9.647, 52.7785) (-9.6021, 52.9878) knots 0 0 0 1 2 2 2
  line L53 (-9.6021, 52.9878) -> (-9.4377, 52.9878)
  line L54 (-0.9655, 48.4378) -> (-0.8159, 48.4079)
  line L55 (-0.8159, 48.4079) -> (-1.3392, 46.7483)
  line L56 (-1.3392, 46.7483) -> (-6.0588, 46.7483)
  line L57 (-6.0588, 46.7483) -> (-6.0588, 46.9128)
  line L58 (-6.0588, 46.9128) -> (-5.8295, 46.9128)
  spline S47 degree 2 poles (-5.8295, 46.9128) (-5.4458, 46.9128) (-5.2813, 47.1669) knots 0 0 0 1 1 1
  spline S48 degree 2 poles (-5.2813, 47.1669) (-5.1866, 47.3065) (-5.1866, 47.8297) knots 0 0 0 1 1 1
  line L59 (-5.1866, 47.8297) -> (-5.1866, 51.7668)
  spline S49 degree 2 poles (-5.1866, 51.7668) (-5.1866, 52.34) (-5.3112, 52.4845) knots 0 0 0 1 1 1
  spline S50 degree 2 poles (-5.3112, 52.4845) (-5.4856, 52.6838) (-5.8295, 52.6838) knots 0 0 0 1 1 1
  line L60 (-5.8295, 52.6838) -> (-6.0588, 52.6838)
  line L61 (-6.0588, 52.6838) -> (-6.0588, 52.8483)
  line L62 (-6.0588, 52.8483) -> (-3.3028, 52.8483)
  line L63 (-3.3028, 52.8483) -> (-3.3028, 52.6838)
  spline S51 degree 2 poles (-3.3028, 52.6838) (-3.7912, 52.6888) (-4.1799, 52.4994) (-4.3244, 52.2104) (-4.3244, 51.6672) knots 0 0 0 1 2 3 3 3
  line L64 (-4.3244, 51.6672) -> (-4.3244, 47.8347)
  spline S52 degree 2 poles (-4.3244, 47.8347) (-4.3244, 47.461) (-4.2547, 47.3214) knots 0 0 0 1 1 1
  spline S53 degree 2 poles (-4.2547, 47.3214) (-4.1999, 47.2267) (-3.9756, 47.137) (-3.3825, 47.137) knots 0 0 0 1 2 2 2
  line L65 (-3.3825, 47.137) -> (-2.939, 47.137)
  spline S54 degree 2 poles (-2.939, 47.137) (-2.2363, 47.137) (-1.6682, 47.3463) (-1.1997, 47.8696) (-0.9655, 48.4378) knots 0 0 0 1 2 3 3 3
  spline S55 degree 2 poles (1.9998, 47.3463) (1.3669, 46.8529) (1.2024, 46.7782) knots 0 0 0 1 1 1
  spline S56 degree 2 poles (1.2024, 46.7782) (0.9632, 46.6636) (0.6891, 46.6636) knots 0 0 0 1 1 1
  spline S57 degree 2 poles (0.6891, 46.6636) (0.2605, 46.6636) (-0.2927, 47.2467) (-0.2927, 47.7251) knots 0 0 0 1 2 2 2
  spline S58 degree 2 poles (-0.2927, 47.7251) (-0.2927, 48.0241) (-0.1581, 48.2484) knots 0 0 0 1 1 1
  spline S59 degree 2 poles (-0.1581, 48.2484) (0.0263, 48.5524) (0.9383, 49.0906) (1.9998, 49.4793) knots 0 0 0 1 2 2 2
  line L66 (1.9998, 49.4793) -> (1.9998, 49.6388)
  spline S60 degree 2 poles (1.9998, 49.6388) (1.9998, 50.2568) (1.6111, 50.7153) (1.2373, 50.7153) knots 0 0 0 1 2 2 2
  spline S61 degree 2 poles (1.2373, 50.7153) (0.9582, 50.7153) (0.7888, 50.5608) knots 0 0 0 1 1 1
  spline S62 degree 2 poles (0.7888, 50.5608) (0.6193, 50.4113) (0.6193, 50.2119) knots 0 0 0 1 1 1
  line L67 (0.6193, 50.2119) -> (0.6293, 49.9528)
  spline S63 degree 2 poles (0.6293, 49.9528) (0.6293, 49.7435) (0.415, 49.5192) (0.2456, 49.5192) knots 0 0 0 1 2 2 2
  spline S64 degree 2 poles (0.2456, 49.5192) (0.0811, 49.5192) (-0.1332, 49.7534) (-0.1332, 49.9578) knots 0 0 0 1 2 2 2
  spline S65 degree 2 poles (-0.1332, 49.9578) (-0.1332, 50.3415) (0.6592, 50.9894) (1.3719, 50.9894) knots 0 0 0 1 2 2 2
  spline S66 degree 2 poles (1.3719, 50.9894) (1.9201, 50.9894) (2.2689, 50.805) knots 0 0 0 1 1 1
  spline S67 degree 2 poles (2.2689, 50.805) (2.5381, 50.6654) (2.6626, 50.3714) knots 0 0 0 1 1 1
  spline S68 degree 2 poles (2.6626, 50.3714) (2.7424, 50.177) (2.7424, 49.579) knots 0 0 0 1 1 1
  line L68 (2.7424, 49.579) -> (2.7424, 48.1786)
  spline S69 degree 2 poles (2.7424, 48.1786) (2.7424, 47.5905) (2.7872, 47.3264) (2.8919, 47.2367) (2.9567, 47.2367) knots 0 0 0 1 2 3 3 3
  spline S70 degree 2 poles (2.9567, 47.2367) (3.0314, 47.2367) (3.0863, 47.2666) knots 0 0 0 1 1 1
  spline S71 degree 2 poles (3.0863, 47.2666) (3.1809, 47.3264) (3.4501, 47.5955) knots 0 0 0 1 1 1
  line L69 (3.4501, 47.5955) -> (3.4501, 47.3463)
  spline S72 degree 2 poles (3.4501, 47.3463) (2.9467, 46.6686) (2.4882, 46.6686) knots 0 0 0 1 1 1
  spline S73 degree 2 poles (2.4882, 46.6686) (2.264, 46.6686) (2.0048, 46.9726) (1.9998, 47.3463) knots 0 0 0 1 2 2 2
  line L70 (1.9998, 47.6354) -> (1.9998, 49.2052)
  spline S74 degree 2 poles (1.9998, 49.2052) (1.322, 48.9361) (1.1227, 48.8215) knots 0 0 0 1 1 1
  spline S75 degree 2 poles (1.1227, 48.8215) (0.7689, 48.6271) (0.4649, 48.1936) (0.4649, 47.9394) knots 0 0 0 1 2 2 2
  spline S76 degree 2 poles (0.4649, 47.9394) (0.4649, 47.6154) (0.8486, 47.1869) (1.1028, 47.1869) knots 0 0 0 1 2 2 2
  spline S77 degree 2 poles (1.1028, 47.1869) (1.4417, 47.1869) (1.9998, 47.6354) knots 0 0 0 1 1 1
  spline S78 degree 2 poles (4.8903, 50.1521) (5.4884, 50.9894) (6.1761, 50.9894) knots 0 0 0 1 1 1
  spline S79 degree 2 poles (6.1761, 50.9894) (6.8091, 50.9894) (7.751, 49.9079) (7.751, 48.966) knots 0 0 0 1 2 2 2
  spline S80 degree 2 poles (7.751, 48.966) (7.751, 47.8696) (7.0233, 47.1968) knots 0 0 0 1 1 1
  spline S81 degree 2 poles (7.0233, 47.1968) (6.4004, 46.6237) (5.6279, 46.6237) knots 0 0 0 1 1 1
  spline S82 degree 2 poles (5.6279, 46.6237) (5.2691, 46.6237) (4.5315, 46.8829) (4.1428, 47.147) knots 0 0 0 1 2 2 2
  line L71 (4.1428, 47.147) -> (4.1428, 51.413)
  spline S83 degree 2 poles (4.1428, 51.413) (4.1428, 52.1107) (4.073, 52.4346) (3.9335, 52.5493) (3.8238, 52.5493) knots 0 0 0 1 2 3 3 3
  spline S84 degree 2 poles (3.8238, 52.5493) (3.6992, 52.5493) (3.5099, 52.4795) knots 0 0 0 1 1 1
  line L72 (3.5099, 52.4795) -> (3.4451, 52.644)
  line L73 (3.4451, 52.644) -> (4.686, 53.1473)
  line L74 (4.686, 53.1473) -> (4.8903, 53.1473)
  line L75 (4.8903, 53.1473) -> (4.8903, 50.1521)
  line L76 (4.8903, 49.8681) -> (4.8903, 47.4061)
  spline S85 degree 2 poles (4.8903, 47.4061) (5.1196, 47.1819) (5.608, 46.9526) (5.8622, 46.9526) knots 0 0 0 1 2 2 2
  spline S86 degree 2 poles (5.8622, 46.9526) (6.2708, 46.9526) (6.9735, 47.8497) (6.9735, 48.7069) knots 0 0 0 1 2 2 2
  spline S87 degree 2 poles (6.9735, 48.7069) (6.9735, 49.4993) (6.2708, 50.3465) (5.8223, 50.3465) knots 0 0 0 1 2 2 2
  spline S88 degree 2 poles (5.8223, 50.3465) (5.5831, 50.3465) (5.3488, 50.2269) knots 0 0 0 1 1 1
  spline S89 degree 2 poles (5.3488, 50.2269) (5.1694, 50.1372) (4.8903, 49.8681) knots 0 0 0 1 1 1
  line L77 (-24.1096, 39.3479) -> (-24.1096, 38.71)
  line L78 (-24.1096, 38.71) -> (-24.9269, 38.71)
  line L79 (-24.9269, 38.71) -> (-24.9269, 37.1003)
  line L80 (-24.9269, 37.1003) -> (-25.6695, 37.1003)
  line L81 (-25.6695, 37.1003) -> (-25.6695, 38.71)
  line L82 (-25.6695, 38.71) -> (-28.256, 38.71)
  line L83 (-28.256, 38.71) -> (-28.256, 39.2831)
  line L84 (-28.256, 39.2831) -> (-25.4203, 43.3249)
  line L85 (-25.4203, 43.3249) -> (-24.9269, 43.3249)
  line L86 (-24.9269, 43.3249) -> (-24.9269, 39.3479)
  line L87 (-24.9269, 39.3479) -> (-24.1096, 39.3479)
  line L88 (-25.6695, 39.3479) -> (-25.6695, 42.378)
  line L89 (-25.6695, 42.378) -> (-27.8124, 39.3479)
  line L90 (-27.8124, 39.3479) -> (-25.6695, 39.3479)
  line L91 (-21.2141, 43.4993) -> (-23.4218, 36.9757)
  line L92 (-23.4218, 36.9757) -> (-23.7807, 36.9757)
  line L93 (-23.7807, 36.9757) -> (-21.5729, 43.4993)
  line L94 (-21.5729, 43.4993) -> (-21.2141, 43.4993)
  line L95 (-17.0029, 38.2714) -> (-17.4315, 37.1003)
  line L96 (-17.4315, 37.1003) -> (-21.0297, 37.1003)
  line L97 (-21.0297, 37.1003) -> (-21.0297, 37.2647)
  spline S90 degree 2 poles (-21.0297, 37.2647) (-19.4399, 38.715) (-18.1441, 40.549) (-18.1441, 41.3115) knots 0 0 0 1 2 2 2
  spline S91 degree 2 poles (-18.1441, 41.3115) (-18.1441, 41.8896) (-18.8568, 42.6371) (-19.3502, 42.6371) knots 0 0 0 1 2 2 2
  spline S92 degree 2 poles (-19.3502, 42.6371) (-19.8037, 42.6371) (-20.5164, 42.1089) (-20.6908, 41.6005) knots 0 0 0 1 2 2 2
  line L98 (-20.6908, 41.6005) -> (-20.8552, 41.6005)
  spline S93 degree 2 poles (-20.8552, 41.6005) (-20.7406, 42.4328) (-19.8137, 43.3249) (-19.1159, 43.3249) knots 0 0 0 1 2 2 2
  spline S94 degree 2 poles (-19.1159, 43.3249) (-18.3734, 43.3249) (-17.3766, 42.373) (-17.3766, 41.7251) knots 0 0 0 1 2 2 2
  spline S95 degree 2 poles (-17.3766, 41.7251) (-17.3766, 41.2616) (-17.5909, 40.7981) knots 0 0 0 1 1 1
  spline S96 degree 2 poles (-17.5909, 40.7981) (-17.9249, 40.0705) (-18.6724, 39.2532) knots 0 0 0 1 1 1
  spline S97 degree 2 poles (-18.6724, 39.2532) (-19.7937, 38.0322) (-20.0728, 37.778) knots 0 0 0 1 1 1
  line L99 (-20.0728, 37.778) -> (-18.478, 37.778)
  spline S98 degree 2 poles (-18.478, 37.778) (-17.9896, 37.778) (-17.6009, 37.8478) (-17.2869, 38.0721) (-17.1673, 38.2714) knots 0 0 0 1 2 3 3 3
  line L100 (-17.1673, 38.2714) -> (-17.0029, 38.2714)
  line L101 (-14.0426, 43.4993) -> (-16.2503, 36.9757)
  line L102 (-16.2503, 36.9757) -> (-16.6092, 36.9757)
  line L103 (-16.6092, 36.9757) -> (-14.4014, 43.4993)
  line L104 (-14.4014, 43.4993) -> (-14.0426, 43.4993)
  line L105 (-9.8314, 38.2714) -> (-10.26, 37.1003)
  line L106 (-10.26, 37.1003) -> (-13.8582, 37.1003)
  line L107 (-13.8582, 37.1003) -> (-13.8582, 37.2647)
  spline S99 degree 2 poles (-13.8582, 37.2647) (-12.2684, 38.715) (-10.9726, 40.549) (-10.9726, 41.3115) knots 0 0 0 1 2 2 2
  spline S100 degree 2 poles (-10.9726, 41.3115) (-10.9726, 41.8896) (-11.6853, 42.6371) (-12.1787, 42.6371) knots 0 0 0 1 2 2 2
  spline S101 degree 2 poles (-12.1787, 42.6371) (-12.6322, 42.6371) (-13.3449, 42.1089) (-13.5193, 41.6005) knots 0 0 0 1 2 2 2
  line L108 (-13.5193, 41.6005) -> (-13.6838, 41.6005)
  spline S102 degree 2 poles (-13.6838, 41.6005) (-13.5691, 42.4328) (-12.6422, 43.3249) (-11.9445, 43.3249) knots 0 0 0 1 2 2 2
  spline S103 degree 2 poles (-11.9445, 43.3249) (-11.2019, 43.3249) (-10.2052, 42.373) (-10.2052, 41.7251) knots 0 0 0 1 2 2 2
  spline S104 degree 2 poles (-10.2052, 41.7251) (-10.2052, 41.2616) (-10.4195, 40.7981) knots 0 0 0 1 1 1
  spline S105 degree 2 poles (-10.4195, 40.7981) (-10.7534, 40.0705) (-11.5009, 39.2532) knots 0 0 0 1 1 1
  spline S106 degree 2 poles (-11.5009, 39.2532) (-12.6222, 38.0322) (-12.9013, 37.778) knots 0 0 0 1 1 1
  line L109 (-12.9013, 37.778) -> (-11.3066, 37.778)
  spline S107 degree 2 poles (-11.3066, 37.778) (-10.8182, 37.778) (-10.4294, 37.8478) (-10.1155, 38.0721) (-9.9958, 38.2714) knots 0 0 0 1 2 3 3 3
  line L110 (-9.9958, 38.2714) -> (-9.8314, 38.2714)
  spline S108 degree 2 poles (-9.1137, 40.1154) (-9.1137, 41.157) (-8.4858, 42.662) (-7.9625, 43.0308) knots 0 0 0 1 2 2 2
  spline S109 degree 2 poles (-7.9625, 43.0308) (-7.5588, 43.3249) (-7.1253, 43.3249) knots 0 0 0 1 1 1
  spline S110 degree 2 poles (-7.1253, 43.3249) (-6.4226, 43.3249) (-5.8644, 42.6122) knots 0 0 0 1 1 1
  spline S111 degree 2 poles (-5.8644, 42.6122) (-5.1667, 41.7251) (-5.1667, 40.2101) knots 0 0 0 1 1 1
  spline S112 degree 2 poles (-5.1667, 40.2101) (-5.1667, 39.1486) (-5.7797, 37.6634) (-6.7266, 36.9956) (-7.1701, 36.9956) knots 0 0 0 1 2 3 3 3
  spline S113 degree 2 poles (-7.1701, 36.9956) (-8.0423, 36.9956) (-8.6253, 38.0272) knots 0 0 0 1 1 1
  spline S114 degree 2 poles (-8.6253, 38.0272) (-9.1137, 38.8944) (-9.1137, 40.1154) knots 0 0 0 1 1 1
  spline S115 degree 2 poles (-8.2316, 40.0008) (-8.2316, 38.7449) (-7.9226, 37.9475) knots 0 0 0 1 1 1
  spline S116 degree 2 poles (-7.9226, 37.9475) (-7.6635, 37.2797) (-7.1552, 37.2797) knots 0 0 0 1 1 1
  spline S117 degree 2 poles (-7.1552, 37.2797) (-6.911, 37.2797) (-6.3927, 37.7133) (-6.2581, 38.2266) knots 0 0 0 1 2 2 2
  spline S118 degree 2 poles (-6.2581, 38.2266) (-6.0488, 38.999) (-6.0488, 40.4044) knots 0 0 0 1 1 1
  spline S119 degree 2 poles (-6.0488, 40.4044) (-6.0488, 41.451) (-6.2631, 42.1437) knots 0 0 0 1 1 1
  spline S120 degree 2 poles (-6.2631, 42.1437) (-6.4275, 42.662) (-6.6817, 42.8763) knots 0 0 0 1 1 1
  spline S121 degree 2 poles (-6.6817, 42.8763) (-6.8661, 43.0258) (-7.1302, 43.0258) knots 0 0 0 1 1 1
  spline S122 degree 2 poles (-7.1302, 43.0258) (-7.4342, 43.0258) (-7.6735, 42.7517) knots 0 0 0 1 1 1
  spline S123 degree 2 poles (-7.6735, 42.7517) (-7.9974, 42.378) (-8.2316, 40.7782) (-8.2316, 40.0008) knots 0 0 0 1 2 2 2
  line L111 (-0.6116, 38.2714) -> (-1.0402, 37.1003)
  line L112 (-1.0402, 37.1003) -> (-4.6384, 37.1003)
  line L113 (-4.6384, 37.1003) -> (-4.6384, 37.2647)
  spline S124 degree 2 poles (-4.6384, 37.2647) (-3.0486, 38.715) (-1.7529, 40.549) (-1.7529, 41.3115) knots 0 0 0 1 2 2 2
  spline S125 degree 2 poles (-1.7529, 41.3115) (-1.7529, 41.8896) (-2.4655, 42.6371) (-2.9589, 42.6371) knots 0 0 0 1 2 2 2
  spline S126 degree 2 poles (-2.9589, 42.6371) (-3.4124, 42.6371) (-4.1251, 42.1089) (-4.2995, 41.6005) knots 0 0 0 1 2 2 2
  line L114 (-4.2995, 41.6005) -> (-4.464, 41.6005)
  spline S127 degree 2 poles (-4.464, 41.6005) (-4.3494, 42.4328) (-3.4224, 43.3249) (-2.7247, 43.3249) knots 0 0 0 1 2 2 2
  spline S128 degree 2 poles (-2.7247, 43.3249) (-1.9821, 43.3249) (-0.9854, 42.373) (-0.9854, 41.7251) knots 0 0 0 1 2 2 2
  spline S129 degree 2 poles (-0.9854, 41.7251) (-0.9854, 41.2616) (-1.1997, 40.7981) knots 0 0 0 1 1 1
  spline S130 degree 2 poles (-1.1997, 40.7981) (-1.5336, 40.0705) (-2.2811, 39.2532) knots 0 0 0 1 1 1
  spline S131 degree 2 poles (-2.2811, 39.2532) (-3.4025, 38.0322) (-3.6816, 37.778) knots 0 0 0 1 1 1
  line L115 (-3.6816, 37.778) -> (-2.0868, 37.778)
  spline S132 degree 2 poles (-2.0868, 37.778) (-1.5984, 37.778) (-1.2097, 37.8478) (-0.8957, 38.0721) (-0.7761, 38.2714) knots 0 0 0 1 2 3 3 3
  line L116 (-0.7761, 38.2714) -> (-0.6116, 38.2714)
  line L117 (3.9086, 43.3249) -> (3.9086, 43.1604)
  spline S133 degree 2 poles (3.9086, 43.1604) (3.3155, 43.1006) (2.558, 42.7468) (1.8254, 42.0191) (1.342, 41.1221) (1.1775, 40.5041) knots 0 0 0 1 2 3 4 4 4
  spline S134 degree 2 poles (1.1775, 40.5041) (1.8304, 40.9526) (2.4832, 40.9526) knots 0 0 0 1 1 1
  spline S135 degree 2 poles (2.4832, 40.9526) (3.1062, 40.9526) (4.0282, 39.9459) (4.0282, 39.1535) knots 0 0 0 1 2 2 2
  spline S136 degree 2 poles (4.0282, 39.1535) (4.0282, 38.391) (3.5647, 37.7581) knots 0 0 0 1 1 1
  spline S137 degree 2 poles (3.5647, 37.7581) (3.0065, 36.9956) (2.0845, 36.9956) knots 0 0 0 1 1 1
  spline S138 degree 2 poles (2.0845, 36.9956) (1.4616, 36.9956) (1.023, 37.4093) knots 0 0 0 1 1 1
  spline S139 degree 2 poles (1.023, 37.4093) (0.1658, 38.2116) (0.1658, 39.4974) knots 0 0 0 1 1 1
  spline S140 degree 2 poles (0.1658, 39.4974) (0.1658, 40.3147) (0.8237, 41.7899) (2.0447, 42.9312) (3.166, 43.3249) (3.6494, 43.3249) knots 0 0 0 1 2 3 4 4 4
  line L118 (3.6494, 43.3249) -> (3.9086, 43.3249)
  spline S141 degree 2 poles (1.1028, 40.1752) (1.023, 39.5722) (1.023, 39.1984) knots 0 0 0 1 1 1
  spline S142 degree 2 poles (1.023, 39.1984) (1.023, 38.7698) (1.342, 37.7581) (1.6559, 37.4591) knots 0 0 0 1 2 2 2
  spline S143 degree 2 poles (1.6559, 37.4591) (1.8902, 37.2498) (2.2191, 37.2498) knots 0 0 0 1 1 1
  spline S144 degree 2 poles (2.2191, 37.2498) (2.6078, 37.2498) (3.2258, 37.9874) (3.2258, 38.6701) knots 0 0 0 1 2 2 2
  spline S145 degree 2 poles (3.2258, 38.6701) (3.2258, 39.4376) (2.6128, 40.5589) (2.0497, 40.5589) knots 0 0 0 1 2 2 2
  spline S146 degree 2 poles (2.0497, 40.5589) (1.8802, 40.5589) (1.4865, 40.4144) (1.1028, 40.1752) knots 0 0 0 1 2 2 2
  point P0 (0, 0)
  constraints: 2 other
extrude "Extrusion16" cut sketch "Sketch15" against normal blind 4
sketch "Sketch16" plane through (-93.3464, 39, 62.7) normal (0, 0, 1) x (1, 0, 0)
  line L0 (6.6464, 0) -> (6.6464, -24) projected
  line L1 (160.0464, -24) -> (160.0464, 0) projected
  line L2 (166.6929, 0) -> (166.6929, -32) projected
  line L3 (0, 0) -> (166.6929, 0) projected
  line L4 (0, -32) -> (0, 0) projected
  line L5 (166.6929, -32) -> (0, -32) projected
  line L6 (160.0464, 0) -> (6.6464, 0) projected
  line L7 (6.6464, -24) -> (160.0464, -24) projected
  line L8 (6.6464, -12) -> (45.8464, -12) construction
  arc A0 (40.3464, -12) -> (45.8464, -17.5) centre (45.8464, -12) ccw
  arc A1 (120.8464, -17.5) -> (126.3464, -12) centre (120.8464, -12) ccw
  line L9 (40.3464, -12) -> (40.3464, 0)
  line L10 (40.3464, 0) -> (51.3464, 0)
  line L11 (115.3464, 0) -> (126.3464, 0)
  line L12 (126.3464, -12) -> (126.3464, 0)
  line L13 (45.8464, -17.5) -> (120.8464, -17.5)
  line L14 (40.3464, 0) -> (126.3464, 0)
  line L15 (40.3464, 0) -> (126.3464, 0)
  point P0 (93.3464, -39)
  point P1 (65.3464, -7.5)
  point P2 (76.3464, -7.5)
  point P3 (90.8464, -7.5)
  point P4 (100.8464, -7.5)
  point P5 (126.3464, 0)
  point P6 (40.3464, 0)
  point P7 (40.3464, 0)
  point P8 (51.3464, 0)
  point P9 (115.3464, 0)
  point P10 (126.3464, 0)
  dimension "d241" = 153.4
  dimension "d242" = 39.2
  dimension "d243" = 11
  dimension "d249" = 11
  constraints: 16 end point, 5 point on line, 4 point on circle, 2 centre point, 2 collinear, 2 perpendicular, 2 tangent, 1 coincident, 1 horizontal, 1 midpoint
  measures "d241" distance between parallel lines of L1 L0
  measures "d242" distance of L8.start L8.end
  measures "d243" diameter of A0
  measures "d249" diameter of A1
extrude "Extrusion17" cut sketch "Sketch16" against normal through all contours L3 L12 A1 L13 A0 L9
ref_plane "Work Plane4" through (66.7, 15, 47.7) normal (0, 0, -1) x (-1, 0, 0)
sketch "Sketch21" plane through (66.7, 15, 47.7) normal (0, 0, -1) x (-1, 0, 0)
  line L0 (7.228, 0) -> (0, 0) construction
  line L1 (0, 0) -> (0, 16) construction
  line L2 (0, 0) -> (0, 24) construction
  arc A0 (0, 16) -> (0, 24) centre (-8.2956, 20) ccw
  line L3 (0, 24) -> (0, 16)
  point P0 (66.7, -15)
  dimension "d263" = 16
  constraints: 4 end point, 2 point on circle, 1 centre point, 1 collinear, 1 point on line
  measures "d263" distance of L0.end L1.end
extrude "Extrusion19" add sketch "Sketch21" along normal mid plane 3
ref_plane "Work Plane5" through (-10, 15, -57.7) normal (-1, 0, 0) x (0, 0, 1)
ref_plane "Work Plane6" through (66.7, 15, 0) normal (0, 0, -1) x (-1, 0, 0)
mirror "Mirror3" about plane through (-10, 15, -57.7) normal (-1, 0, 0) of "Extrusion19"
mirror "Mirror4" about plane through (66.7, 15, 0) normal (0, 0, -1) of "Extrusion19", "Mirror3"
sketch "Sketch22" plane through (0, 15, 0) normal (0, 1, 0) x (1, 0, 0)
  line L0 (55.857, -25.95) -> (55.857, 25.95) projected
  line L1 (-75.857, 25.95) -> (-75.857, -25.95) projected
  line L2 (30.1507, 0) -> (55.857, 0) construction
  circle A0 centre (43.0038, 0) radius 3.25
  point P0 (0, 0)
  dimension "d268" = 6.5
  constraints: 2 end point, 2 midpoint, 1 centre point
  measures "d268" diameter of A0